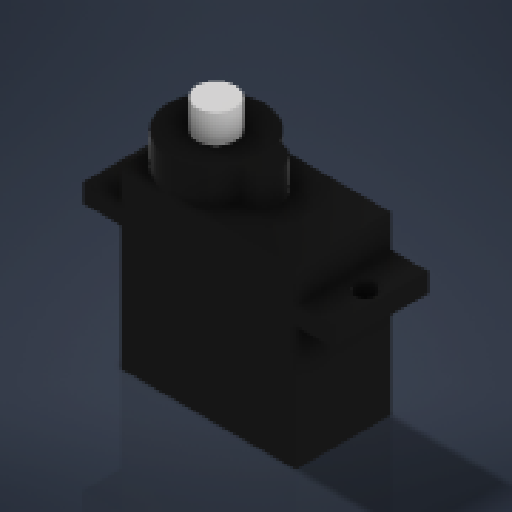
# Autodesk Inventor part: Motor_V1
Saved by Autodesk Inventor 2024.1 (Build 281209000, 209)
## iProperties
Created: 2023-05-18
Part Number: Motor_V1
Material: Acetal Resin, Black
Document SubType Name: Modeling
Designer: jaege
Density: 1.425 g/cm^3
Appearance: Smooth - Black
Author: jaege
Autodesk Inventor part; units mm, degrees
ref_plane "YZ Plane" through (0, 0, 0) normal (1, 0, 0) x (0, 1, 0)
ref_plane "XZ Plane" through (0, 0, 0) normal (0, 1, 0) x (-1, 0, 0)
ref_plane "XY Plane" through (0, 0, 0) normal (0, 0, 1) x (1, 0, 0)
sketch "Sketch1" plane through (0, 0, 0) normal (0, 1, 0) x (-1, 0, 0)
  line L0 (11.25, 6.1) -> (-11.25, 6.1)
  line L1 (-11.25, 6.1) -> (-11.25, -6.1)
  line L2 (-11.25, -6.1) -> (11.25, -6.1)
  line L3 (11.25, -6.1) -> (11.25, 6.1)
  line L4 (11.25, 6.1) -> (-11.25, -6.1) construction
  line L5 (-11.25, 6.1) -> (11.25, -6.1) construction
  point P0 (0, 0)
  dimension "d0" = 22.5
  dimension "d1" = 12.2
  constraints: 12 end point, 2 midpoint, 2 parallel, 1 horizontal, 1 perpendicular
  measures "d0" distance of L2.end L1.end
  measures "d1" distance of L1.end L0.end
extrude "Extrusion1" add sketch "Sketch1" along normal blind 16
sketch "Sketch2" plane through (0, 16, 0) normal (0, 1, 0) x (1, 0, 0)
  line L0 (11.25, -6.1) -> (11.25, 6.1) construction
  line L1 (11.25, 6.1) -> (-11.25, 6.1) projected
  line L2 (-11.25, 6.1) -> (-11.25, -6.1) construction
  line L3 (-11.25, -6.1) -> (11.25, -6.1) projected
  line L4 (11.25, 6.1) -> (-11.25, 6.1) projected
  line L5 (-11.25, 6.1) -> (-16.1, 6.1)
  line L6 (-16.1, 6.1) -> (-16.1, -6.1)
  line L7 (-11.25, 6.1) -> (-11.25, -6.1) projected
  line L8 (-16.1, -6.1) -> (-11.25, -6.1)
  line L9 (11.25, -6.1) -> (11.25, 6.1) projected
  line L10 (11.25, -6.1) -> (16.1, -6.1)
  line L11 (16.1, -6.1) -> (16.1, 6.1)
  line L12 (16.1, 6.1) -> (11.25, 6.1)
  circle A0 centre (-14.1, 0) radius 1.4
  circle A1 centre (14.1, 0) radius 1.4
  line L13 (-11.25, -6.1) -> (11.25, -6.1) construction
  line L14 (0, -6.1) -> (0, 6.1) construction
  point P0 (0, 0)
  dimension "d5" = 32.2
  dimension "d6" = 2.8
  dimension "d7" = 2.8
  dimension "d8" = 31
  constraints: 14 end point, 3 horizontal, 2 centre point, 2 horizontal alignment, 2 midpoint, 2 vertical, 1 collinear, 1 perpendicular, 1 symmetric about line
  measures "d5" distance between parallel lines of L11 L6
  measures "d6" diameter of A0
  measures "d7" diameter of A1
extrude "Extrusion2" add sketch "Sketch2" along normal blind 2.5
sketch "Sketch3" plane through (0, 18.5, 0) normal (0, 1, 0) x (1, 0, 0)
  line L0 (11.25, -6.1) -> (11.25, 6.1) projected
  line L1 (-11.25, -6.1) -> (11.25, -6.1) projected
  line L2 (-11.25, 6.1) -> (-11.25, -6.1) projected
  line L3 (11.25, 6.1) -> (-11.25, 6.1) projected
  point P0 (0, 0)
extrude "Extrusion3" add sketch "Sketch3" along normal blind 4.2
sketch "Sketch4" plane through (0, 22.7, 0) normal (0, 1, 0) x (1, 0, 0)
  arc A0 (-5.15, 6.1) -> (0.295, -2.75) centre (-5.15, 0) ccw
  arc A1 (0.2987, 2.7426) -> (0.5, -2.75) centre (0.5, 0) ccw construction
  line L0 (11.25, 6.1) -> (-11.25, 6.1) projected
  line L1 (-11.25, 6.1) -> (-11.25, -6.1) projected
  line L2 (-11.25, -6.1) -> (11.25, -6.1) projected
  line L3 (11.25, -6.1) -> (11.25, 6.1) projected
  line L4 (0.295, 2.75) -> (0.5, 2.75)
  line L5 (0.5, -2.75) -> (0.295, -2.75)
  arc A2 (0.5, 2.75) -> (0.2987, 2.7426) centre (0.5, 0) ccw
  arc A3 (0.295, 2.75) -> (-5.15, 6.1) centre (-5.15, 0) ccw
  arc A4 (0.295, -2.75) -> (0.295, 2.75) centre (-5.15, 0) ccw construction
  arc A5 (0.5, -2.75) -> (0.5, 2.75) centre (0.5, 0) ccw
  point P0 (0, 0)
  dimension "d13" = 5.5
  dimension "d14" = 14.5
  constraints: 14 point on circle, 10 tangent, 6 centre point, 4 end point, 2 horizontal, 1 horizontal alignment, 1 point on line
  measures "d13" diameter of A1
extrude "Extrusion4" add sketch "Sketch4" along normal blind 4 contours A3 L4 A5 L5 A0
sketch "Sketch5" plane through (0, 26.7, 0) normal (0, 1, 0) x (1, 0, 0)
  circle A0 centre (-5.15, 0) radius 2.5
  arc A1 (0.295, 2.75) -> (0.295, -2.75) centre (-5.15, 0) ccw projected
  point P0 (0, 0)
  dimension "d17" = 5
  constraints: 1 centre point, 1 concentric
  measures "d17" diameter of A0
extrude "Extrusion5" add sketch "Sketch5" along normal blind 3.7
body "Solid1"
